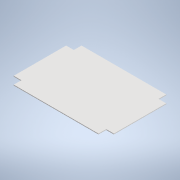
# Autodesk Inventor part: Pieza35
Saved by Autodesk Inventor 2022.2 (Build 262287000, 287)
## iProperties
Created: 2022-02-11
Part Number: Pieza35
Material: Aluminio 6061
Document SubType Name: Modeling
Designer: USUARIO
Density: 2.7 g/cm^3
Appearance: Aluminio - Plano
Author: USUARIO
Autodesk Inventor part; units mm, degrees
ref_plane "YZ Plane" through (0, 0, 0) normal (1, 0, 0) x (0, 1, 0)
ref_plane "XZ Plane" through (0, 0, 0) normal (0, 1, 0) x (-1, 0, 0)
ref_plane "XY Plane" through (0, 0, 0) normal (0, 0, 1) x (1, 0, 0)
sketch "Boceto2" plane through (0, 0, 0) normal (0, 1, 0) x (-1, 0, 0)
  line L0 (385.3386, 43.2382) -> (385.3386, -6.7618)
  line L1 (385.3386, -6.7618) -> (435.3386, -6.7618)
  line L2 (385.3386, -446.7618) -> (385.3386, -396.7618)
  line L3 (385.3386, -396.7618) -> (435.3386, -396.7618)
  line L4 (-164.6614, 43.2382) -> (-164.6614, -6.7618)
  line L5 (-164.6614, -6.7618) -> (-214.6614, -6.7618)
  line L6 (-164.6614, -446.7618) -> (-164.6614, -396.7618)
  line L7 (-164.6614, -396.7618) -> (-214.6614, -396.7618)
  line L8 (385.3386, 43.2382) -> (-164.6614, 43.2382)
  line L9 (435.3386, -396.7618) -> (435.3386, -6.7618)
  line L10 (-214.6614, -6.7618) -> (-214.6614, -396.7618)
  line L11 (-164.6614, -446.7618) -> (-214.6614, -446.7618)
  line L12 (-214.6614, -446.7618) -> (-214.6614, -596.7618)
  line L13 (-214.6614, -596.7618) -> (435.3386, -596.7618)
  line L14 (435.3386, -596.7618) -> (435.3386, -446.7618)
  line L15 (435.3386, -446.7618) -> (385.3386, -446.7618)
  point P0 (0, 0)
  dimension "d15" = 50
  dimension "d16" = 50
  dimension "d17" = 50
  dimension "d18" = 50
  dimension "d19" = 50
  dimension "d20" = 50
  dimension "d21" = 50
  dimension "d22" = 50
  dimension "d25" = 50
  dimension "d26" = 150
  dimension "d27" = 650
  dimension "d28" = 150
  constraints: 32 end point, 4 perpendicular, 2 horizontal, 1 parallel, 1 point on line
  measures "d15" distance of L1.end L0.end
  measures "d16" distance of L0.end L0.start
  measures "d17" distance of L2.end L3.end
  measures "d18" distance of L2.start L2.end
  measures "d19" distance of L4.end L5.end
  measures "d20" distance of L4.start L4.end
  measures "d21" distance of L7.end L6.end
  measures "d22" distance of L6.end L6.start
  measures "d25" distance of L6.start L11.end
  measures "d26" distance of L11.end L12.end
  measures "d27" distance of L12.end L13.end
  measures "d28" distance of L13.end L14.end
extrude "Extrusión2" add sketch "Boceto2" along normal blind 5
sketch "Boceto3" plane through (0, 5, 0) normal (0, 1, 0) x (1, 0, 0)
  arc A0 (-61.5546, 521.7618) -> (-74.0546, 521.7618) centre (-67.8046, 521.7618) ccw projected
  arc A1 (103.4454, 521.7618) -> (90.9454, 521.7618) centre (97.1954, 521.7618) ccw projected
  arc A2 (90.9454, 241.7618) -> (103.4454, 241.7618) centre (97.1954, 241.7618) ccw projected
  arc A3 (-74.0546, 241.7618) -> (-61.5546, 241.7618) centre (-67.8046, 241.7618) ccw projected
  circle A4 centre (-67.8046, 241.7618) radius 6.25
  circle A5 centre (97.1954, 241.7618) radius 6.25
  circle A6 centre (97.1954, 521.7618) radius 6.25
  circle A7 centre (-67.8046, 521.7618) radius 6.25
  point P0 (0, 0)
  constraints: 4 coincident, 1 centre point, 1 concentric, 9 other
extrude "Extrusión3" cut sketch "Boceto3" against normal through all
